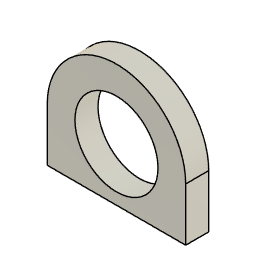
KS5N-IG36P_Mount2 (Autodesk Fusion 360 design; units mm, degrees)
Autodesk Fusion 360 part; units mm, degrees
note: some values were not read from the file. Chosen so that the rebuilt part matches the saved one: a direction; which face or edge a step refers to; how an offset face is resized.
sketch "スケッチ1" plane through (0, 0, 0) normal (0, 0, 1) x (1, 0, 0)
  line L0 (30, 5) -> (-30, 5)
  line L1 (-30, 5) -> (-30, -5)
  line L2 (-30, -5) -> (30, -5)
  line L3 (30, -5) -> (30, 5)
  line L4 (30, 5) -> (-30, -5) construction
  line L5 (-30, 5) -> (30, -5) construction
  dimension "d1" = 60
  dimension "d2" = 10
  constraint horizontal L0
  constraint perpendicular L0 L1
  constraint parallel L0 L2
  constraint parallel L1 L3
  constraint coincident L4 origin
  constraint coincident L5 origin
  measures "d1" distance of L1.end L2.end
  measures "d2" distance of L0.end L1.end
extrude "押し出し1" add sketch "スケッチ1" along normal blind 55
sketch "スケッチ2" plane through (0, -5, 0) normal (0, -1, 0) x (1, 0, 0)
  line L0 (-30, 0) -> (30, 0)
  line L1 (30, 0) -> (30, 55)
  line L2 (30, 55) -> (-30, 55)
  line L3 (-30, 55) -> (-30, 0)
  line L4 (0, 0) -> (0, 25)
  circle A0 centre (0, 25) radius 11
  circle A1 centre (0, 25) radius 18
  dimension "d5" = 25
  dimension "d6" = 22
  dimension "d7" = 36
  constraint coincident L4.start origin
  constraint perpendicular L0 L4
  constraint coincident L4.end A0.centre
  constraint concentric A0 A1
  measures "d5" distance of L4.start L4.end
  measures "d6" diameter of A0
  measures "d7" diameter of A1
extrude "押し出し2" cut sketch "スケッチ2" against normal blind 10 contours A0
extrude "押し出し3" cut sketch "スケッチ2" against normal blind 2 contours A1
sketch "スケッチ3" plane through (0, 0, 0) normal (0, 0, -1) x (1, 0, 0)
  line L0 (30, -5) -> (30, 5)
  line L1 (30, 5) -> (-30, 5)
  line L2 (-30, 5) -> (-30, -5)
  line L3 (-30, -5) -> (30, -5)
  line L4 (0, 0) -> (15, 0)
  line L5 (0, 0) -> (-15, 0)
  circle A0 centre (-15, 0) radius 2
  circle A1 centre (15, 0) radius 2
  dimension "d12" = 15
  dimension "d13" = 15
  dimension "d14" = 4
  dimension "d15" = 4
  constraint coincident L4.start L5.start
  constraint parallel L3 L4
  constraint parallel L4 L5
  constraint coincident L5.end A0.centre
  constraint coincident L4.end A1.centre
  measures "d12" distance of L4.start L4.end
  measures "d13" distance of L4.start L5.end
  measures "d14" diameter of A0
  measures "d15" diameter of A1
extrude "押し出し4" cut sketch "スケッチ3" against normal blind 10 contours A0 | A1
thread "ねじ1" "ISO Metric profile 3.0 M3x0.5 6H" major diameter 3.086 minor diameter 2.529 pitch 0.5 angle 60 resizes the face on face at (-13.0025, 0.0997, 6.6667)
thread "ねじ2" "ISO Metric profile 3.0 M3x0.5 6H" major diameter 3.086 minor diameter 2.529 pitch 0.5 angle 60 resizes the face on face at (16.9975, 0.0997, 6.6667)
fillet "フィレット1" radius 30 2 edges at (30, 0, 55) (-30, 0, 55)
extrude "押し出し6" add 1 faces at (15.5587, -3, 23.5593) along direction (0, -1, 0) blind 2
sketch "スケッチ5" plane through (0, -5, 0) normal (0, -1, 0) x (1, 0, 0)
  circle A0 centre (0, 25) radius 11
  arc A1 (30, 25) -> (-30, 25) centre (0, 25) ccw
  line L0 (-30, 25) -> (-30, 0)
  line L1 (-30, 0) -> (30, 0)
  line L2 (30, 0) -> (30, 25)
  circle A2 centre (0, 25) radius 18
  dimension "d38" = 36
  constraint concentric A0 A2
  measures "d38" diameter of A2
extrude "押し出し7" cut sketch "スケッチ5" against normal blind 10 contours A2
extrude "押し出し8" cut 1 faces at (-25.4215, 0, 0) along direction (0, 0, 1) blind 2
